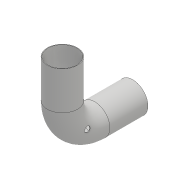
# Autodesk Inventor part: knee 90
Saved by Autodesk Inventor 2018 (Build 220112000, 112)
## iProperties
Created: 2019-12-18
Part Number: knee 90
Material: Generic
Document SubType Name: Modeling
Designer: Ibnu
Density: 1 g/cm^3
Appearance: Default
Author: Ibnu
Autodesk Inventor part; units mm, degrees
ref_plane "Work Plane1" through (0, 0, 61.5) normal (0, 0, 1) x (1, 0, 0)
sketch "Sketch1" plane through (0, 0, 61.5) normal (0, 0, 1) x (1, 0, 0)
  circle A0 centre (0, 0) radius 13.25
  dimension "d1" = 26.5
  constraints: 1 centre point, 1 coincident
  measures "d1" diameter of A0
ref_plane "Work Plane2" through (0, 61.5, 0) normal (0, 1, 0) x (-1, 0, 0)
sketch "Sketch2" plane through (0, 61.5, 0) normal (0, 1, 0) x (-1, 0, 0)
  circle A0 centre (0, 0) radius 13.25
  dimension "d3" = 26.5
  constraints: 1 centre point, 1 coincident
  measures "d3" diameter of A0
sketch "Sketch3" plane through (0, 0, 0) normal (1, 0, 0) x (0, 1, 0)
  line L0 (13.25, 61.5) -> (-13.25, 61.5) construction
  line L1 (61.5, -13.25) -> (61.5, 13.25) construction
  line L2 (0, -28.2) -> (0, 76.45) construction
  line L3 (-28.2, 0) -> (76.45, 0) construction
  line L4 (0, 0) -> (0, 61.5)
  line L5 (0, 0) -> (61.5, 0)
  line L6 (61.5, 13.25) -> (28.25, 13.25)
  line L7 (13.25, 28.25) -> (13.25, 61.5)
  arc A0 (13.25, 28.25) -> (28.25, 13.25) centre (28.25, 28.25) ccw
  dimension "d4" = 15
  constraints: 8 end point, 2 midpoint, 2 point on circle, 2 point on line, 2 tangent, 1 centre point, 1 other
  measures "d4" radius of A0
sweep "Sweep1" add profiles "Sketch1" path "Sketch3" path curves L7 A0 L6
shell "Shell1" thickness 0.5 removed faces 2 at (0.1548, 61.5, -7.494) at (-0.404, -5.4414, 61.5)
ref_plane "Work Plane3" through (26.75, 0, 0) normal (1, 0, 0) x (0, 1, 0)
sketch "Sketch4" plane through (26.75, 0, 0) normal (1, 0, 0) x (0, 1, 0)
  circle A0 centre (8.6449, 8.6449) radius 2.5
  point P0 (0, 0)
  constraints: 1 centre point
extrude "Extrusion1" cut sketch "Sketch4" against normal through all
body "Solid1"
